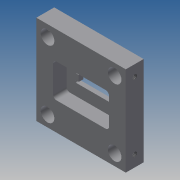
# Autodesk Inventor part: HolderStart
Saved by Autodesk Inventor 2015 (Build 190159000, 159)
## iProperties
Created: 2014-07-11
Part Number: HolderStart
Material: Generic
Document SubType Name: Modeling
Designer: jad211
Density: 1 g/cm^3
Appearance: Default
Author: jad211
Autodesk Inventor part; units mm, degrees
ref_plane "YZ Plane" through (0, 0, 0) normal (1, 0, 0) x (0, 1, 0)
ref_plane "XZ Plane" through (0, 0, 0) normal (0, 1, 0) x (-1, 0, 0)
ref_plane "XY Plane" through (0, 0, 0) normal (0, 0, 1) x (1, 0, 0)
sketch "Sketch1" plane through (0, 0, 0) normal (0, 1, 0) x (-1, 0, 0)
  line L0 (20, 20) -> (20, -20)
  line L1 (20, -20) -> (-20, -20)
  line L2 (-20, -20) -> (-20, 20)
  line L3 (-20, 20) -> (20, 20)
  line L4 (-15, 15) -> (-15, -15) construction
  line L5 (-15, -15) -> (15, -15) construction
  line L6 (15, -15) -> (15, 15) construction
  line L7 (15, 15) -> (-15, 15) construction
  circle A0 centre (15, 15) radius 3.05
  circle A1 centre (15, -15) radius 3.05
  circle A2 centre (-15, -15) radius 3.05
  circle A3 centre (-15, 15) radius 3.05
  line L8 (0, 0) -> (-18.5703, 0) construction
  line L9 (0, 0) -> (0, 25.6262) construction
  line L10 (0, 0) -> (-18.05, 0) construction
  line L11 (8, 2.3333) -> (-8, 2.3333)
  line L12 (-8.5, 1.8333) -> (-8.5, 1.8333)
  line L13 (8.5, 1.8333) -> (8.5, 1.8333)
  line L14 (8.5, 2.3333) -> (-8.5, 3.0056) construction
  line L15 (-8.5, 2.3333) -> (8.5, 3.0548) construction
  arc A4 (8.5, 1.8333) -> (8, 2.3333) centre (8, 1.8333) ccw
  arc A5 (8, 1.3333) -> (8.5, 1.8333) centre (8, 1.8333) ccw
  arc A6 (-8.5, 1.8333) -> (-8, 1.3333) centre (-8, 1.8333) ccw
  arc A7 (-8, 2.3333) -> (-8.5, 1.8333) centre (-8, 1.8333) ccw
  line L16 (-8.5, -1.8333) -> (-8.5, -1.8333)
  line L17 (-8, -2.3333) -> (8, -2.3333)
  line L18 (8.5, -1.8333) -> (8.5, -1.8333)
  line L19 (8.5, -0.691) -> (-8.5, -2.3333) construction
  line L20 (-8.5, -0.6827) -> (8.5, -2.3333) construction
  arc A8 (8.5, -1.8333) -> (8.0002, -1.3333) centre (8, -1.8333) ccw
  arc A9 (8, -2.3333) -> (8.5, -1.8333) centre (8, -1.8333) ccw
  arc A10 (-8.5, -1.8333) -> (-8, -2.3333) centre (-8, -1.8333) ccw
  arc A11 (-8, -1.3333) -> (-8.5, -1.8333) centre (-8, -1.8333) ccw
  line L21 (8, 1.3333) -> (7, 1.3333)
  line L22 (7, 1.3333) -> (7, -1.3333)
  line L23 (7, -1.3333) -> (8.0002, -1.3333)
  line L24 (-8, 1.3333) -> (-7, 1.3333)
  line L25 (-7, 1.3333) -> (-7, -1.3333)
  line L26 (-7, -1.3333) -> (-8, -1.3333)
  point P0 (0, -12.01)
  point P1 (-0.3001, 2.6813)
  point P2 (0, 2.694)
  point P3 (0.0215, -1.5101)
  point P4 (0, -1.508)
  point P5 (0, -1.5122)
  dimension "d0" = 40
  dimension "d1" = 40
  dimension "d2" = 30
  dimension "d53" = 20
  dimension "d114" = 17
  dimension "d117" = 0.5
  dimension "d140" = 17
  dimension "d142" = 0.5
  dimension "d146" = 14
  dimension "d147" = 7
  dimension "d150" = 1.3333
  dimension "d151" = 1.3333
  dimension "d152" = 2.3333
  dimension "d153" = 2.3333
  constraints: 54 end point, 19 point on line, 16 point on circle, 13 perpendicular, 12 centre point, 12 tangent, 9 equal radius, 7 coincident, 3 horizontal, 3 midpoint, 2 collinear, 2 vertical, 1 parallel
  measures "d0" distance of L0.end L1.end
  measures "d1" distance of L0.start L0.end
  measures "d2" distance of L5.end L6.end
  measures "d53" distance from line of L8.start L1
  measures "d114" distance between parallel lines of L12 L13
  measures "d117" radius of A4
  measures "d140" distance between parallel lines of L16 L18
  measures "d142" radius of A8
  measures "d146" distance between parallel lines of L25 L22
  measures "d147" distance from line of L25 L8.start
  measures "d150" distance from line of L8.start L26
  measures "d151" distance from line of L24 L8.start
  measures "d152" distance from line of L8.start L11
  measures "d153" distance from line of L8.start L17
extrude "Extrusion15" add sketch "Sketch1" along normal blind 5
sketch "Sketch11" plane through (0, 0, 0) normal (0, -1, 0) x (1, 0, 0)
  line L0 (-11, -7.5) -> (11, -7.5)
  line L1 (12.5, -6) -> (12.5, 6)
  line L2 (11, 7.5) -> (-11, 7.5)
  line L3 (-12.5, 6) -> (-12.5, -6)
  line L4 (-12.5, -7.5) -> (12.5, 7.5) construction
  line L5 (12.5, -7.5) -> (-12.5, 7.5) construction
  arc A0 (-11, 7.5) -> (-12.5, 6) centre (-11, 6) ccw
  arc A1 (-12.5, -6) -> (-11, -7.5) centre (-11, -6) ccw
  arc A2 (11, -7.5) -> (12.5, -6) centre (11, -6) ccw
  arc A3 (12.5, 6) -> (11, 7.5) centre (11, 6) ccw
  point P0 (0, 0)
  dimension "d154" = 15
  dimension "d155" = 25
  dimension "d156" = 1.5
  constraints: 12 end point, 8 point on circle, 8 point on line, 8 tangent, 4 centre point, 3 equal radius, 3 perpendicular, 2 midpoint, 1 horizontal
  measures "d154" distance of L5.start L4.end
  measures "d155" distance of L4.end L5.end
  measures "d156" radius of A0
extrude "Extrusion16" cut sketch "Sketch11" against normal blind 3
sketch "Sketch14" plane through (0, 0, 0) normal (0, -1, 0) x (1, 0, 0)
  arc A0 (-12.5, -6) -> (-11, -7.5) centre (-11, -6) ccw projected
  line L0 (-12.5, -6) -> (-12.5, 6) projected
  arc A1 (-11, 7.5) -> (-12.5, 6) centre (-11, 6) ccw projected
  line L1 (-11, 7.5) -> (11, 7.5) projected
  arc A2 (12.5, 6) -> (11, 7.5) centre (11, 6) ccw projected
  line L2 (12.5, 6) -> (12.5, -6) projected
  arc A3 (11, -7.5) -> (12.5, -6) centre (11, -6) ccw projected
  line L3 (11, -7.5) -> (-11, -7.5) projected
  circle A4 centre (15, 15) radius 3.05 projected
  circle A5 centre (15, -15) radius 3.05 projected
  circle A6 centre (-15, -15) radius 3.05 projected
  circle A7 centre (-15, 15) radius 3.05 projected
  line L4 (-20, 20) -> (-20, -20) projected
  line L5 (-20, -20) -> (20, -20) projected
  line L6 (20, -20) -> (20, 20) projected
  line L7 (20, 20) -> (-20, 20) projected
  point P0 (0, 0)
extrude "Extrusion17" add sketch "Sketch14" along normal blind 3
sketch "Sketch12" plane through (20, 0, 20) normal (1, 0, 0) x (0, 0, -1)
  line L0 (40, 5) -> (40, -3) projected
  line L1 (0, 5) -> (40, 5) projected
  line L2 (0, 5) -> (0, -3) projected
  line L3 (40, -3) -> (0, -3) projected
  point P0 (20, 0)
  point P1 (5, 1)
  point P2 (35, 1)
  dimension "d163" = 5
  dimension "d164" = 5
  dimension "d165" = 4
  dimension "d166" = 4
  measures "d163" distance from line of L2 point (5, 1)
  measures "d164" distance from line of L0 point (35, 1)
  measures "d165" distance from line of L1 point (5, 1)
  measures "d166" distance from line of L1 point (35, 1)
hole "Hole1" at (20, 1, 15) at (20, 1, -15) direction (-1, 0, 0) diameter 2.013 depth 5 tip angle 118 thread size "M2.5x0.45" class "6H" standard "ISO Metric profile"
sketch "Sketch13" plane through (-20, 0, -20) normal (-1, 0, 0) x (0, 0, 1)
  line L0 (40, -3) -> (40, 5) projected
  line L1 (0, 5) -> (40, 5) projected
  line L2 (0, 5) -> (0, -3) projected
  circle A0 centre (35, 1) radius 1.0065 projected
  circle A1 centre (5, 1) radius 1.0065 projected
  line L3 (40, -3) -> (0, -3) projected
  point P0 (20, 0)
  point P1 (33.9935, 1)
  point P2 (3.9935, 1)
  constraints: 2 coincident, 2 horizontal alignment, 2 other
hole "Hole2" at (-20, 1, 15) at (-20, 1, -15) direction (1, 0, 0) diameter 2.013 depth 5 tip angle 118 thread size "M2.5x0.45" class "6H" standard "ISO Metric profile"
equation "\"d1\" = d0"
body "Solid4"
